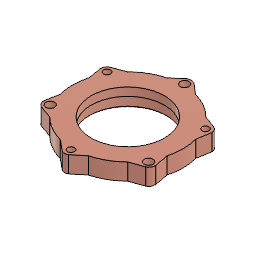
Cover (Autodesk Fusion 360 design; units mm, degrees)
Autodesk Fusion 360 part; units mm, degrees
sketch "Sketch2" plane through (0, 0, 0) normal (0, 0, 1) x (1, 0, 0)
  circle A0 centre (0, 0) radius 34
  circle A1 centre (0, 0) radius 23.5
  circle A2 centre (0, 0) radius 31
  circle A3 centre (0, 0) radius 25.5
  circle A4 centre (0, 0) radius 22.5
  line L0 (0, 0) -> (0, 35) construction
  circle A5 centre (0, 35) radius 1.65
  circle A6 centre (0, 35) radius 4.15
  circle A7 centre (0, 35) radius 2.7
  line L1 (0, 0) -> (19.7922, 0) construction
  line L2 (0, 0) -> (0, -35) construction
  circle A8 centre (0, -35) radius 2.15
  circle A9 centre (0, -35) radius 3.95
  circle A10 centre (-30.3109, -17.5) radius 1.65
  circle A11 centre (-30.3109, -17.5) radius 2.7
  circle A12 centre (-30.3109, -17.5) radius 4.15
  circle A13 centre (30.3109, 17.5) radius 2.15
  circle A14 centre (30.3109, 17.5) radius 3.95
  circle A15 centre (30.3109, -17.5) radius 1.65
  circle A16 centre (30.3109, -17.5) radius 2.7
  circle A17 centre (30.3109, -17.5) radius 4.15
  circle A18 centre (-30.3109, 17.5) radius 2.15
  circle A19 centre (-30.3109, 17.5) radius 3.95
  dimension "d19" = 68
  dimension "d21" = 47
  dimension "d29" = 62
  dimension "d36" = 2
  dimension "d104" = 35
  dimension "d105" = 3.3
  dimension "d106" = 2.5
  dimension "d107" = 5.4
  dimension "d108" = 4.3
  dimension "d109" = 1.8
  dimension "d111" = 360
  constraint coincident A0.centre A1.centre
  constraint concentric A0 A1
  constraint concentric A0 A2
  constraint vertical L0
  constraint coincident L0.end A5.centre
  constraint concentric A5 A7
  constraint horizontal L1
  constraint symmetric A0.centre L1 A1.centre
  constraint symmetric L0.end L1 L2.end
  constraint coincident L2.end A8.centre
  measures "d19" diameter of A0
  measures "d21" diameter of A1
  measures "d29" diameter of A2
  measures "d104" distance of A0.centre L0.end
  measures "d105" diameter of A5
  measures "d107" diameter of A7
  measures "d108" diameter of A8
extrude "main" add sketch "Sketch2" along normal blind 5 contours A0 A2 A6 A14 A17 | A0 A13 A14 | A0 A13 A14 | A0 A16 A17 | A0 A2 A16 A17 | A0 A15 A16 | A0 A15 A16 | A2 A6 A12 A17 | A2 A17 | A0 A2 A6 A7 | A0 A6 A7 | A0 A2 A9 A12 A17 | A0 A5 A7 | A0 A5 A7 | A2 A6 | A0 A8 A9 | A0 A8 A9 | A0 A2 A11 A12 | A2 A12 | A0 A2 A6 A12 A19 | A0 A18 A19 | A0 A18 A19 | A0 A11 A12 | A0 A10 A11 | A0 A10 A11 | A1 | A3
extrude "outer ring and heat insert holders" add sketch "Sketch2" against normal blind 5.3 contours A0 A2 A6 A14 A17 | A0 A13 A14 | A0 A13 A14 | A0 A16 A17 | A0 A2 A16 A17 | A0 A15 A16 | A0 A15 A16 | A0 A2 A6 A7 | A0 A6 A7 | A0 A2 A9 A12 A17 | A0 A5 A7 | A0 A5 A7 | A0 A8 A9 | A0 A8 A9 | A0 A2 A11 A12 | A0 A2 A6 A12 A19 | A0 A18 A19 | A0 A18 A19 | A0 A11 A12 | A0 A10 A11 | A0 A10 A11
extrude "bearing mount" add sketch "Sketch2" against normal blind 7 contours A3
extrude "Extrude9" cut sketch "Sketch2" against normal blind 4 from surface at 5 contours A0 A15 A16 | A0 A15 A16 | A0 A15 | A0 A15 | A0 A5 A7 | A0 A5 A7 | A0 A5 | A0 A5 | A0 A10 A11 | A0 A10 A11 | A0 A10 | A0 A10
fillet "Fillet3" radius 1 1 edges at (-21.9097, -8.498, -7)
chamfer "Chamfer3" distance 5 angle 45 1 edges at (-23.7743, -9.2212, 0)
chamfer "Chamfer4" distance 5 angle 45 12 edges at (-27.2627, -20.3162, -0.15) (-31.2257, -13.4521, -0.15) (-3.7606, -33.7914, -0.15) (3.7606, -33.7914, -0.15) (27.2627, -20.3162, -0.15) (31.2257, -13.4521, -0.15) (31.1445, 13.639, -0.15) (27.3839, 20.1524, -0.15) (3.963, 33.7683, -0.15) (-3.963, 33.7683, -0.15) (-27.3839, 20.1524, -0.15) (-31.1445, 13.639, -0.15)
equation "gear_ratio = 6"
equation "gear_Ns = if(is_Nema_17 == 1; 12; 15)"
equation "gear_Nr = ( gear_ratio - 1 ) * gear_Ns"
equation "gear_OD = ( gear_Nr * module * diameter_scale ) + 8 mm"
equation "thickness = 2 mm"
equation "m3_pilot = 3.3 mm"
equation "d19 = gear_OD"
equation "bearing_OD = ( if(gear_ratio == 6; 47.1; if(gear_ratio == 7; 52; if(gear_ratio == 8; 58; if(gear_ratio == 9; 65; if(gear_ratio == 10; 72; 0))))) ) * 1 mm"
equation "d21 = bearing_OD - bearing_mount_clearance"
equation "d26 = thickness + m3_head_height"
equation "height = 5.3 mm"
equation "d29 = gear_OD - wall_thickness"
equation "wall_thickness = 6 mm"
equation "d31 = -height"
equation "bearing_mount_clearance = 0.1 mm"
equation "bearing_width = ( if(gear_ratio < 10; 7; 9) ) * 1 mm"
equation "bearing_mount_wall_thickness = 2 mm"
equation "d36 = bearing_mount_wall_thickness"
equation "d37 = -bearing_width"
equation "bearing_mount_lip = 1 mm"
equation "bearing_mount_lip_height = 2 mm"
equation "d46 = -bearing_mount_lip"
equation "m3_inserts_diameter = 4.3 mm"
equation "m3_inserts_wall_thickness = 1.8 mm"
equation "m3_head_diameter = 5.2 mm + 0.2 mm"
equation "m3_head_height = 3 mm"
equation "m3_chamfer = 1 mm"
equation "module = 1"
equation "helix_angle = 0 deg"
equation "diameter_scale = ( 1 / cos(helix_angle) ) * 1 mm"
equation "d104 = ( gear_OD / 2 ) + 1 mm"
equation "d105 = m3_pilot"
equation "d107 = m3_head_diameter"
equation "d108 = m3_inserts_diameter"
equation "d109 = m3_inserts_wall_thickness"
equation "d113 = -m3_head_height - m3_chamfer"
equation "is_Nema_17 = 1"
